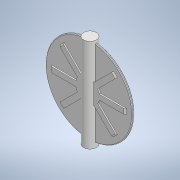
# Autodesk Inventor part: Butterfly Valve
Saved by Autodesk Inventor 2020.2 (Build 242310000, 310)
## iProperties
Created: 2020-04-12
Part Number: Butterfly Valve
Material: Generic
Document SubType Name: Modeling
Designer: Josiah
Density: 1 g/cm^3
Appearance: Default
Author: Josiah
Autodesk Inventor part; units mm, degrees
ref_plane "YZ Plane" through (0, 0, 0) normal (1, 0, 0) x (0, 1, 0)
ref_plane "XZ Plane" through (0, 0, 0) normal (0, 1, 0) x (-1, 0, 0)
ref_plane "XY Plane" through (0, 0, 0) normal (0, 0, 1) x (1, 0, 0)
sketch "Sketch1" plane through (0, 0, 0) normal (0, 0, 1) x (1, 0, 0)
  circle A0 centre (0, 0) radius 100
  dimension "d0" = 200
  constraints: 1 centre point, 1 coincident
  measures "d0" diameter of A0
extrude "Extrusion1" add sketch "Sketch1" along normal mid plane 5
sketch "Sketch2" plane through (0, 0, 0) normal (0, 1, 0) x (-1, 0, 0)
  circle A0 centre (0, 0) radius 14.8
  line L0 (-100, -2.5) -> (100, -2.5) projected
  line L1 (100, 2.5) -> (-100, 2.5) projected
  dimension "d3" = 29.6
  dimension "d23" = 5
  dimension "d24" = 2.5
  dimension "d25" = 0
  constraints: 1 centre point
  measures "d3" diameter of A0
  measures "d23" distance between parallel lines of L0 L1
  measures "d24" distance from line of L0 A0.centre
  measures "d25" distance of point (0, 0) A0.centre
extrude "Extrusion2" add sketch "Sketch2" along normal blind 105.5 and the other way blind 109.5
sketch "Sketch3" plane through (0, 0, 2.5) normal (0, 0, 1) x (1, 0, 0)
  circle A0 centre (0, 0) radius 27.5 construction
  arc A1 (-14.5873, 98.9303) -> (-14.5873, -98.9303) centre (0, 0) ccw projected
  line L0 (26.8375, 6) -> (99.8198, 6)
  line L1 (26.8375, -6) -> (99.8198, -6)
  arc A2 (14.5873, -98.9303) -> (14.5873, 98.9303) centre (0, 0) ccw projected
  line L2 (86.8375, 6) -> (86.8375, -6)
  arc A3 (23.2196, -14.7343) -> (26.8375, -6) centre (0, 0) ccw
  line L3 (0, 0) -> (23.2196, -14.7343) construction
  line L4 (0, 0) -> (26.8375, -6) construction
  line L5 (23.2196, 14.7343) -> (74.8259, 66.3406)
  line L6 (14.7343, 23.2196) -> (66.3406, 74.8259)
  line L7 (57.1607, 65.646) -> (65.646, 57.1607)
  arc A4 (26.8375, 6) -> (23.2196, 14.7343) centre (0, 0) ccw
  line L8 (6, 26.8375) -> (6, 99.8198)
  line L9 (-6, 26.8375) -> (-6, 99.8198)
  line L10 (-6, 86.8375) -> (6, 86.8375)
  arc A5 (14.7343, 23.2196) -> (6, 26.8375) centre (0, 0) ccw
  line L11 (-14.7343, 23.2196) -> (-66.3406, 74.8259)
  line L12 (-23.2196, 14.7343) -> (-74.8259, 66.3406)
  line L13 (-65.646, 57.1607) -> (-57.1607, 65.646)
  arc A6 (-6, 26.8375) -> (-14.7343, 23.2196) centre (0, 0) ccw
  line L14 (-26.8375, 6) -> (-99.8198, 6)
  line L15 (-26.8375, -6) -> (-99.8198, -6)
  line L16 (-86.8375, -6) -> (-86.8375, 6)
  arc A7 (-23.2196, 14.7343) -> (-26.8375, 6) centre (0, 0) ccw
  line L17 (-23.2196, -14.7343) -> (-74.8259, -66.3406)
  line L18 (-14.7343, -23.2196) -> (-66.3406, -74.8259)
  line L19 (-57.1607, -65.646) -> (-65.646, -57.1607)
  arc A8 (-26.8375, -6) -> (-23.2196, -14.7343) centre (0, 0) ccw
  line L20 (-6, -26.8375) -> (-6, -99.8198)
  line L21 (6, -26.8375) -> (6, -99.8198)
  line L22 (6, -86.8375) -> (-6, -86.8375)
  arc A9 (-14.7343, -23.2196) -> (-6, -26.8375) centre (0, 0) ccw
  line L23 (14.7343, -23.2196) -> (66.3406, -74.8259)
  line L24 (23.2196, -14.7343) -> (74.8259, -66.3406)
  line L25 (65.646, -57.1607) -> (57.1607, -65.646)
  arc A10 (6, -26.8375) -> (14.7343, -23.2196) centre (0, 0) ccw
  point P0 (-23.2196, 14.7343)
  point P1 (-26.8375, -6)
  point P2 (17.0679, -21.5624)
  point P3 (26.8375, 6)
  point P4 (-14.7343, -23.2196)
  point P5 (6, -26.8375)
  point P6 (23.2196, -14.7343)
  dimension "innerDia" = 55
  dimension "spokeThickness" = 12
  dimension "d10" = 6
  dimension "d12" = 60
  dimension "d13" = 19.796
  dimension "d16" = 360
  constraints: 52 end point, 20 point on circle, 16 point on line, 9 centre point, 2 coincident, 1 horizontal, 1 vertical, 97 other
  measures "innerDia" diameter of A0
  measures "spokeThickness" distance between parallel lines of L0 L1
  measures "d10" distance from line of point (0, 0) L1
  measures "d12" distance from line of L2 L0.start
  measures "d13" angle of L3 L4
extrude "Extrusion3" add sketch "Sketch3" along normal blind 3 contours L11 A6 L9 L10 L8 A5 L6 L7 L5 A4 L0 L2 L1 A3 L24 L25 L23 A10 L21 L22 L20 A9 L18 L19 L17 A8 L15 L16 L14 A7 L12 L13
chamfer "Chamfer1" distance 3 angle 45 6 edges at (-61.4034, 61.4034, 5.5) (61.4034, 61.4034, 5.5) (86.8375, 0, 5.5) (-61.4034, -61.4034, 5.5) (-86.8375, 0, 5.5) (61.4034, -61.4034, 5.5)
mirror "Mirror2" about plane through (0, 0, 0) normal (0, 0, 1) of "Extrusion3", "Chamfer1"
fillet "Fillet2" radius 1.5 4 edges at (-100, 0, 2.5) (-100, 0, -2.5) (100, 0, 2.5) (100, 0, -2.5)
sketch "Sketch6" plane through (0, -109.5, 0) normal (0, -1, 0) x (1, 0, 0)
  arc A0 (2.832, 0.9898) -> (2.0133, -2.2241) centre (0, 0) ccw construction
  line L0 (2.832, 0.9898) -> (2.0133, -2.2241) construction
  arc A1 (3.0404, 0.9979) -> (2.1924, -2.3309) centre (0, 0) ccw
  line L1 (3.0404, 0.9979) -> (2.1924, -2.3309)
  point P0 (0, 0)
  dimension "d33" = 0.2
  constraints: 4 end point, 4 point on circle, 2 centre point, 1 other
  measures "d33" radial gap between concentric circles of A0 A1
extrude "Extrusion5" cut sketch "Sketch6" against normal blind 15
equation "\"d10\" = 0.5 * spokeThickness"
equation "\"toleranceFactor\" = 0.1"
body "Solid1"
